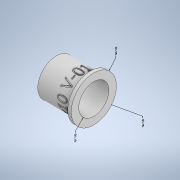
# Autodesk Inventor part: frontPipeDrain-V01
Saved by Autodesk Inventor 2021.1 (Build 251245010, 245A)
## iProperties
Created: 2020-10-20
Part Number: frontPipeDrain-V01
Material: Generic
Document SubType Name: Modeling
Designer: robst
Density: 1 g/cm^3
Appearance: Default
Author: robst
Autodesk Inventor part; units mm, degrees
ref_plane "YZ Plane" through (0, 0, 0) normal (1, 0, 0) x (0, 1, 0)
ref_plane "XZ Plane" through (0, 0, 0) normal (0, 1, 0) x (-1, 0, 0)
sketch "Sketch2" plane through (0, 0, 0) normal (0, 0, 1) x (1, 0, 0)
  line L0 (0, 0) -> (0, 20.955)
  line L1 (0, 20.955) -> (-3.175, 20.955)
  line L2 (-3.175, 20.955) -> (-3.175, 17.145)
  line L3 (-3.175, 17.145) -> (-28.575, 17.145)
  line L4 (-28.575, 17.145) -> (-28.575, 13.97)
  line L5 (-28.575, 13.97) -> (0, 13.97)
  line L6 (-41.91, 0) -> (6.985, 0) projected
  line L7 (-28.575, 13.97) -> (-34.925, 13.97)
  line L8 (-34.925, 13.97) -> (-34.925, 17.145)
  line L9 (-34.925, 17.145) -> (-28.575, 17.145)
  line L10 (-28.575, 17.145) -> (-28.575, 13.97)
  dimension "d0" = 20.955
  dimension "d1" = 13.97
  dimension "d2" = 3.175
  dimension "d3" = 25.4
  dimension "d5" = 17.145
  dimension "d6" = 6.35
  constraints: 20 end point, 6 perpendicular, 2 parallel, 1 collinear, 1 horizontal, 1 point on line, 1 vertical
  measures "d0" distance from line of L0.start L1
  measures "d1" distance from line of L5 L0.start
  measures "d2" distance between parallel lines of L0 L2
  measures "d3" distance from line of L3.end L2
  measures "d5" distance from line of L3 L0.start
  measures "d6" distance between parallel lines of L8 L4
revolve "Revolution1" add sketch "Sketch2" angle 360 about axis through (-10, 0, 0) along (1, 0, 0)
ref_plane "Work Plane1" through (-19.05, 0, 17.145) normal (0, 0, 1) x (1, 0, 0)
sketch "Sketch5" plane through (-19.05, 0, 17.145) normal (0, 0, 1) x (1, 0, 0)
  line L0 (-15.875, 17.145) -> (15.875, 17.145) projected
  line L1 (-15.875, -17.145) -> (15.875, -17.145) projected
  line L2 (15.875, -20.955) -> (15.875, 20.955) projected
  line L3 (6.985, -17.145) -> (6.985, 17.145) construction
  spline S0 degree 2 poles (4.6292, -29.2455) (5.2128, -29.2455) (6.1277, -29.6345) (6.4735, -29.9587) knots 0 0 0 1 2 2 2
  spline S1 degree 2 poles (6.4735, -29.9587) (6.8193, -30.2757) (7.4028, -31.097) (7.6766, -31.5509) knots 0 0 0 1 2 2 2
  line L4 (7.6766, -31.5509) -> (9.0382, -31.5509)
  line L5 (9.0382, -31.5509) -> (9.0382, -32.6171)
  line L6 (9.0382, -32.6171) -> (7.2155, -32.6171)
  spline S2 degree 2 poles (7.2155, -32.6171) (7.0138, -32.2857) (6.4519, -31.3924) (6.2069, -31.1402) knots 0 0 0 1 2 2 2
  spline S3 degree 2 poles (6.2069, -31.1402) (5.8972, -30.8232) (5.1767, -30.463) (4.7157, -30.463) knots 0 0 0 1 2 2 2
  spline S4 degree 2 poles (4.7157, -30.463) (4.0457, -30.463) (3.3829, -31.3131) (3.3829, -31.9903) knots 0 0 0 1 2 2 2
  spline S5 degree 2 poles (3.3829, -31.9903) (3.3829, -32.5883) (3.7791, -33.6401) (3.9953, -33.9715) knots 0 0 0 1 2 2 2
  line L7 (3.9953, -33.9715) -> (3.9953, -34.0363)
  line L8 (3.9953, -34.0363) -> (2.7777, -34.0363)
  spline S6 degree 2 poles (2.7777, -34.0363) (2.6192, -33.6401) (2.3599, -32.4226) (2.3599, -31.875) knots 0 0 0 1 2 2 2
  spline S7 degree 2 poles (2.3599, -31.875) (2.3599, -30.6503) (3.6062, -29.2455) (4.6292, -29.2455) knots 0 0 0 1 2 2 2
  line L9 (11.43, -31.4572) -> (11.43, -32.6675)
  line L10 (11.43, -32.6675) -> (10.1693, -32.6675)
  line L11 (10.1693, -32.6675) -> (10.1693, -31.4572)
  line L12 (10.1693, -31.4572) -> (11.43, -31.4572)
  line L13 (11.43, -26.335) -> (11.43, -27.7614)
  line L14 (11.43, -27.7614) -> (9.7298, -27.7614)
  line L15 (9.7298, -27.7614) -> (9.7298, -26.335)
  line L16 (9.7298, -26.335) -> (11.43, -26.335)
  spline S8 degree 2 poles (4.6292, -19.7504) (5.2128, -19.7504) (6.1277, -20.1394) (6.4735, -20.4636) knots 0 0 0 1 2 2 2
  spline S9 degree 2 poles (6.4735, -20.4636) (6.8193, -20.7806) (7.4028, -21.6018) (7.6766, -22.0557) knots 0 0 0 1 2 2 2
  line L17 (7.6766, -22.0557) -> (9.0382, -22.0557)
  line L18 (9.0382, -22.0557) -> (9.0382, -23.1219)
  line L19 (9.0382, -23.1219) -> (7.2155, -23.1219)
  spline S10 degree 2 poles (7.2155, -23.1219) (7.0138, -22.7905) (6.4519, -21.8972) (6.2069, -21.6451) knots 0 0 0 1 2 2 2
  spline S11 degree 2 poles (6.2069, -21.6451) (5.8972, -21.3281) (5.1767, -20.9679) (4.7157, -20.9679) knots 0 0 0 1 2 2 2
  spline S12 degree 2 poles (4.7157, -20.9679) (4.0457, -20.9679) (3.3829, -21.818) (3.3829, -22.4952) knots 0 0 0 1 2 2 2
  spline S13 degree 2 poles (3.3829, -22.4952) (3.3829, -23.0931) (3.7791, -24.1449) (3.9953, -24.4763) knots 0 0 0 1 2 2 2
  line L20 (3.9953, -24.4763) -> (3.9953, -24.5412)
  line L21 (3.9953, -24.5412) -> (2.7777, -24.5412)
  spline S14 degree 2 poles (2.7777, -24.5412) (2.6192, -24.1449) (2.3599, -22.9274) (2.3599, -22.3799) knots 0 0 0 1 2 2 2
  spline S15 degree 2 poles (2.3599, -22.3799) (2.3599, -21.1552) (3.6062, -19.7504) (4.6292, -19.7504) knots 0 0 0 1 2 2 2
  line L22 (11.43, -21.962) -> (11.43, -23.1724)
  line L23 (11.43, -23.1724) -> (10.1693, -23.1724)
  line L24 (10.1693, -23.1724) -> (10.1693, -21.962)
  line L25 (10.1693, -21.962) -> (11.43, -21.962)
  spline S16 degree 2 poles (4.6292, -13.9582) (5.2128, -13.9582) (6.1277, -14.3472) (6.4735, -14.6714) knots 0 0 0 1 2 2 2
  spline S17 degree 2 poles (6.4735, -14.6714) (6.8193, -14.9884) (7.4028, -15.8096) (7.6766, -16.2635) knots 0 0 0 1 2 2 2
  line L26 (7.6766, -16.2635) -> (9.0382, -16.2635)
  line L27 (9.0382, -16.2635) -> (9.0382, -17.3297)
  line L28 (9.0382, -17.3297) -> (7.2155, -17.3297)
  spline S18 degree 2 poles (7.2155, -17.3297) (7.0138, -16.9983) (6.4519, -16.105) (6.2069, -15.8529) knots 0 0 0 1 2 2 2
  spline S19 degree 2 poles (6.2069, -15.8529) (5.8972, -15.5359) (5.1767, -15.1757) (4.7157, -15.1757) knots 0 0 0 1 2 2 2
  spline S20 degree 2 poles (4.7157, -15.1757) (4.0457, -15.1757) (3.3829, -16.0258) (3.3829, -16.703) knots 0 0 0 1 2 2 2
  spline S21 degree 2 poles (3.3829, -16.703) (3.3829, -17.3009) (3.7791, -18.3527) (3.9953, -18.6841) knots 0 0 0 1 2 2 2
  line L29 (3.9953, -18.6841) -> (3.9953, -18.749)
  line L30 (3.9953, -18.749) -> (2.7777, -18.749)
  spline S22 degree 2 poles (2.7777, -18.749) (2.6192, -18.3527) (2.3599, -17.1352) (2.3599, -16.5877) knots 0 0 0 1 2 2 2
  spline S23 degree 2 poles (2.3599, -16.5877) (2.3599, -15.363) (3.6062, -13.9582) (4.6292, -13.9582) knots 0 0 0 1 2 2 2
  line L31 (11.43, -16.1699) -> (11.43, -17.3802)
  line L32 (11.43, -17.3802) -> (10.1693, -17.3802)
  line L33 (10.1693, -17.3802) -> (10.1693, -16.1699)
  line L34 (10.1693, -16.1699) -> (11.43, -16.1699)
  line L35 (11.43, -7.6113) -> (11.43, -8.9873)
  line L36 (11.43, -8.9873) -> (8.9229, -10.6082)
  line L37 (8.9229, -10.6082) -> (11.43, -12.2724)
  line L38 (11.43, -12.2724) -> (11.43, -13.5475)
  line L39 (11.43, -13.5475) -> (8.1233, -11.235)
  line L40 (8.1233, -11.235) -> (4.7589, -13.5259)
  line L41 (4.7589, -13.5259) -> (4.7589, -12.1499)
  line L42 (4.7589, -12.1499) -> (7.2444, -10.5362)
  line L43 (7.2444, -10.5362) -> (4.7589, -8.8864)
  line L44 (4.7589, -8.8864) -> (4.7589, -7.6113)
  line L45 (4.7589, -7.6113) -> (8.0512, -9.9094)
  line L46 (8.0512, -9.9094) -> (11.43, -7.6113)
  line L47 (11.43, -1.8695) -> (11.43, -6.2064)
  line L48 (11.43, -6.2064) -> (10.5223, -6.2064)
  line L49 (10.5223, -6.2064) -> (10.5223, -4.5927)
  line L50 (10.5223, -4.5927) -> (4.5644, -4.5927)
  line L51 (4.5644, -4.5927) -> (4.5644, -6.2064)
  line L52 (4.5644, -6.2064) -> (3.7503, -6.2064)
  spline S24 degree 2 poles (3.7503, -6.2064) (3.7503, -5.2915) (3.2316, -4.427) (2.5112, -4.3694) knots 0 0 0 1 2 2 2
  line L53 (2.5112, -4.3694) -> (2.5112, -3.4472)
  line L54 (2.5112, -3.4472) -> (10.5223, -3.4472)
  line L55 (10.5223, -3.4472) -> (10.5223, -1.8695)
  line L56 (10.5223, -1.8695) -> (11.43, -1.8695)
  spline S25 degree 2 poles (6.985, 5.2987) (9.3768, 5.2987) (11.6173, 3.9083) (11.6173, 2.4602) knots 0 0 0 1 2 2 2
  spline S26 degree 2 poles (11.6173, 2.4602) (11.6173, 0.9906) (9.3336, -0.3854) (6.9922, -0.3854) knots 0 0 0 1 2 2 2
  spline S27 degree 2 poles (6.9922, -0.3854) (4.586, -0.3854) (2.3599, 1.005) (2.3599, 2.4602) knots 0 0 0 1 2 2 2
  spline S28 degree 2 poles (2.3599, 2.4602) (2.3599, 3.9227) (4.6652, 5.2987) (6.985, 5.2987) knots 0 0 0 1 2 2 2
  spline S29 degree 2 poles (9.6938, 3.7714) (9.2543, 3.9443) (7.8999, 4.0884) (6.985, 4.0884) knots 0 0 0 1 2 2 2
  spline S30 degree 2 poles (6.985, 4.0884) (6.0701, 4.0884) (4.7229, 3.9443) (4.269, 3.7642) knots 0 0 0 1 2 2 2
  spline S31 degree 2 poles (4.269, 3.7642) (3.8151, 3.5841) (3.3469, 2.9573) (3.3469, 2.4602) knots 0 0 0 1 2 2 2
  spline S32 degree 2 poles (3.3469, 2.4602) (3.3469, 1.9631) (3.8151, 1.322) (4.2834, 1.1347) knots 0 0 0 1 2 2 2
  spline S33 degree 2 poles (4.2834, 1.1347) (4.7373, 0.9546) (6.1205, 0.8249) (6.9922, 0.8249) knots 0 0 0 1 2 2 2
  spline S34 degree 2 poles (6.9922, 0.8249) (7.9288, 0.8249) (9.1823, 0.9402) (9.6722, 1.1275) knots 0 0 0 1 2 2 2
  spline S35 degree 2 poles (9.6722, 1.1275) (10.1332, 1.3004) (10.6303, 1.9415) (10.6303, 2.4602) knots 0 0 0 1 2 2 2
  spline S36 degree 2 poles (10.6303, 2.4602) (10.6303, 2.9501) (10.1621, 3.5913) (9.6938, 3.7714) knots 0 0 0 1 2 2 2
  line L57 (2.54, 16.9551) -> (11.43, 13.8933)
  line L58 (11.43, 13.8933) -> (11.43, 12.6182)
  line L59 (11.43, 12.6182) -> (2.54, 9.5564)
  line L60 (2.54, 9.5564) -> (2.54, 10.8243)
  line L61 (2.54, 10.8243) -> (9.9243, 13.2882)
  line L62 (9.9243, 13.2882) -> (2.54, 15.752)
  line L63 (2.54, 15.752) -> (2.54, 16.9551)
  line L64 (8.08, 20.9102) -> (8.08, 17.5459)
  line L65 (8.08, 17.5459) -> (6.9994, 17.5459)
  line L66 (6.9994, 17.5459) -> (6.9994, 20.9102)
  line L67 (6.9994, 20.9102) -> (8.08, 20.9102)
  spline S37 degree 2 poles (6.985, 27.6246) (9.3768, 27.6246) (11.6173, 26.2341) (11.6173, 24.7861) knots 0 0 0 1 2 2 2
  spline S38 degree 2 poles (11.6173, 24.7861) (11.6173, 23.3164) (9.3336, 21.9404) (6.9922, 21.9404) knots 0 0 0 1 2 2 2
  spline S39 degree 2 poles (6.9922, 21.9404) (4.586, 21.9404) (2.3599, 23.3308) (2.3599, 24.7861) knots 0 0 0 1 2 2 2
  spline S40 degree 2 poles (2.3599, 24.7861) (2.3599, 26.2486) (4.6652, 27.6246) (6.985, 27.6246) knots 0 0 0 1 2 2 2
  spline S41 degree 2 poles (9.6938, 26.0973) (9.2543, 26.2702) (7.8999, 26.4143) (6.985, 26.4143) knots 0 0 0 1 2 2 2
  spline S42 degree 2 poles (6.985, 26.4143) (6.0701, 26.4143) (4.7229, 26.2702) (4.269, 26.0901) knots 0 0 0 1 2 2 2
  spline S43 degree 2 poles (4.269, 26.0901) (3.8151, 25.91) (3.3469, 25.2832) (3.3469, 24.7861) knots 0 0 0 1 2 2 2
  spline S44 degree 2 poles (3.3469, 24.7861) (3.3469, 24.289) (3.8151, 23.6478) (4.2834, 23.4605) knots 0 0 0 1 2 2 2
  spline S45 degree 2 poles (4.2834, 23.4605) (4.7373, 23.2804) (6.1205, 23.1507) (6.9922, 23.1507) knots 0 0 0 1 2 2 2
  spline S46 degree 2 poles (6.9922, 23.1507) (7.9288, 23.1507) (9.1823, 23.266) (9.6722, 23.4533) knots 0 0 0 1 2 2 2
  spline S47 degree 2 poles (9.6722, 23.4533) (10.1332, 23.6262) (10.6303, 24.2674) (10.6303, 24.7861) knots 0 0 0 1 2 2 2
  spline S48 degree 2 poles (10.6303, 24.7861) (10.6303, 25.276) (10.1621, 25.9172) (9.6938, 26.0973) knots 0 0 0 1 2 2 2
  line L68 (11.43, 33.7986) -> (11.43, 29.4616)
  line L69 (11.43, 29.4616) -> (10.5223, 29.4616)
  line L70 (10.5223, 29.4616) -> (10.5223, 31.0754)
  line L71 (10.5223, 31.0754) -> (4.5644, 31.0754)
  line L72 (4.5644, 31.0754) -> (4.5644, 29.4616)
  line L73 (4.5644, 29.4616) -> (3.7503, 29.4616)
  spline S49 degree 2 poles (3.7503, 29.4616) (3.7503, 30.3766) (3.2316, 31.2411) (2.5112, 31.2987) knots 0 0 0 1 2 2 2
  line L74 (2.5112, 31.2987) -> (2.5112, 32.2208)
  line L75 (2.5112, 32.2208) -> (10.5223, 32.2208)
  line L76 (10.5223, 32.2208) -> (10.5223, 33.7986)
  line L77 (10.5223, 33.7986) -> (11.43, 33.7986)
  point P0 (19.05, 0)
  dimension "d35" = 8.89
  constraints: 2 end point, 2 point on line, 1 perpendicular, 1 vertical
  measures "d35" distance between parallel lines of L3 L2
emboss "Emboss1" sketch "Sketch5" operation cut depth 1.27 direction (0, 0, -1) wrap yes faces at (-13.7583, 16.923, -2.7503) contours S22 S23 S16 S17 L26 L27 L1 S18 S19 S20 S21 | L1 S21 L29 L30 S22 | L1 L27 L28 S18 | L33 L34 L31 L1 | L1 L31 L32 L33 | S0 S1 L4 L5 L6 S2 S3 S4 S5 L7 L8 S6 S7 | L9 L10 L11 L12 | L13 L14 L15 L16 | S8 S9 L17 L18 L19 S10 S11 S12 S13 L20 L21 S14 S15 | L22 L23 L24 L25 | L35 L36 L37 L38 L39 L40 L41 L42 L43 L44 L45 L46 | L47 L48 L49 L50 L51 L52 S24 L53 L54 L55 L56 | S25 S26 S27 S28 | L57 L58 L59 L60 L61 L62 L63 | L64 L65 L66 L67 | S37 S38 S39 S40 | L68 L69 L70 L71 L72 L73 S49 L74 L75 L76 L77
sketch "Sketch4" plane through (0, 0, 0) normal (0, 0, 1) x (1, 0, 0)
  line L0 (-38.4127, 15.1606) -> (-37.6784, 13.8887)
  line L1 (-37.2516, 13.8887) -> (-36.5173, 15.1606)
  arc A0 (-37.6784, 13.8887) -> (-37.2516, 13.8887) centre (-37.465, 14.0119) ccw
  line L2 (-39.0573, 15.1606) -> (-40.3283, 12.9592)
  line L3 (-35.8727, 15.1606) -> (-33.7873, 11.5486)
  arc A1 (-38.4127, 15.1606) -> (-39.0573, 15.1606) centre (-38.735, 14.9745) ccw
  arc A2 (-35.8727, 15.1606) -> (-36.5173, 15.1606) centre (-36.195, 14.9745) ccw
  line L4 (-38.735, 15.3467) -> (-36.195, 15.3467)
  line L5 (-34.925, -17.145) -> (-34.925, 17.145) construction
  line L6 (-34.925, 0) -> (-40.005, 0) construction
  line L7 (-40.3283, 12.9592) -> (-40.3283, 16.2117) construction
  point P0 (0, 0)
  dimension "d10" = 60
  dimension "d11" = 0.2464
  dimension "d12" = 60
  dimension "d13" = 60
  dimension "d15" = 2.54
  dimension "d16" = 5.08
  dimension "d17" = 1.27
  dimension "d18" = 15.3467
  dimension "d19" = 13.7655
  dimension "d20" = 30
  constraints: 14 end point, 8 point on circle, 6 tangent, 3 centre point, 2 horizontal, 1 equal radius, 1 midpoint, 1 vertical
  measures "d10" angle of L1 L0
  measures "d11" radius of A0
  measures "d12" angle of L0 L2
  measures "d13" angle of L3 L1
  measures "d15" distance of A2.centre A1.centre
  measures "d16" distance from line of L6.end L5
  measures "d17" distance from line of A2.centre L5
  measures "d18" distance between parallel lines of L4 L6
  measures "d19" distance edge to line of A0 L6
  measures "d20" angle of L7 L2
equation "\"d0\" = flangeRadius"
equation "\"d1\" = pipeRadius"
equation "\"d2\" = flangeThickness"
equation "\"d3\" = houseWallThickness"
equation "\"d5\" = houseHoleRadius"
equation "\"d6\" = allowanceForThreadRing"
equation "\"d10\" = threadAngle"
equation "\"d11\" = a1RootRadius"
equation "\"d12\" = threadAngle"
equation "\"d13\" = threadAngle"
equation "\"d15\" = pitch"
equation "\"d16\" = 2 * pitch"
equation "\"d17\" = 0.5 * pitch"
equation "\"d18\" = 0.5 * a1MajorDiameter"
equation "\"d19\" = 0.5 * a1MinorDiameter"
equation "\"d20\" = 0.5 * threadAngle"
equation "\"houseHoleDiameter\" = 34.29"
equation "\"pipeDiameter\" = 27.94"
equation "\"houseHoleRadius\" = 0.5 * houseHoleDiameter"
equation "\"pipeRadius\" = 0.5 * pipeDiameter"
equation "\"houseWallThickness\" = 25.4"
equation "\"allowanceForThreadRing\" = 6.35"
equation "\"threadDepth\" = 15.875"
equation "\"flangeDiameter\" = 41.91"
equation "\"flangeRadius\" = 0.5 * flangeDiameter"
equation "\"a1MajorDiameter\" = 30.69336"
equation "\"a1MinorDiameter\" = 27.53106"
equation "\"a1RootRadius\" = 0.24638"
equation "\"threadAngle\" = 60deg"
equation "\"flangeThickness\" = 3.175"
equation "\"pitch\" = 2.54"
body "Solid1"
